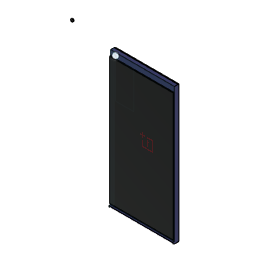
phone v1 (Autodesk Fusion 360 design; units mm, degrees)
Autodesk Fusion 360 part; units mm, degrees
sketch "Sketch1" plane through (0, 0, 0) normal (0, 1, 0) x (1, 0, 0)
  line L0 (-19.0423, -73.6284) -> (-12.0423, -73.6284)
  line L1 (-12.0423, -73.6284) -> (-12.0423, -58.6284)
  line L2 (-12.0423, -58.6284) -> (-19.0423, -58.6284)
  line L3 (-19.0423, -58.6284) -> (-19.0423, -73.6284)
  line L4 (-18.5, -73) -> (-16.5, -73)
  line L5 (-16.5, -73) -> (-16.5, -69)
  line L6 (-16.5, -69) -> (-18.5, -69)
  line L7 (-18.5, -69) -> (-18.5, -73)
  circle A0 centre (-17.5247, -72.1484) radius 0.6603
  circle A1 centre (-17.5247, -70.6133) radius 0.6107
  circle A2 centre (-18, -69.5) radius 0.2531
  circle A3 centre (-17, -69.5) radius 0.2276
  dimension "d1" = 7
  dimension "d2" = 15
  dimension "d3" = 2
  dimension "d4" = 4
  constraint horizontal L0
  constraint vertical L1
  constraint horizontal L2
  constraint vertical L3
  constraint horizontal L4
  constraint vertical L5
  constraint horizontal L6
  constraint vertical L7
  measures "d1" distance of L0.start L0.end
  measures "d2" distance of L0.start L2.end
  measures "d3" distance of L4.start L4.end
  measures "d4" distance of L4.start L6.end
extrude "Extrude1" add sketch "Sketch1" against normal blind 1 contours L0 L1 L2 L3 makes body 1
extrude "Extrude2" add sketch "Sketch1" along normal blind 0.5 separate body contours L4 L5 L6 L7 makes body 2
extrude "Extrude3" add sketch "Sketch1" along normal blind 1 contours A0 bodies 2
extrude "Extrude4" add sketch "Sketch1" along normal blind 0.75 contours A1 bodies 2
extrude "Extrude5" cut 1 faces at (-17.3264, 1, 72.3095) along direction (0, -1, 0) blind 0.25 on bodies 2 bodies 2
extrude "Extrude6" add sketch "Sketch1" along normal blind 0.65 contours A2 | A3 bodies 2
extrude "Extrude7" cut 1 faces at (-15.8615, -1, 62.0856) along direction (0, 1, 0) blind 0.2 on bodies 1 bodies 1
chamfer "Chamfer1" distance 0.1 angle 45 8 edges at (-15.5423, 0, 73.6284) (-19.0423, 0, 66.1284) (-12.0423, 0, 66.1284) (-15.5423, 0, 58.6284) (-16.5, 0.5, 71) (-18.5, 0.5, 71) (-17.5, 0.5, 69) (-17.5, 0.5, 73) 1 faces at (-17.8333, 0.1667, 73) on bodies 1 2
fillet "Fillet1" radius 0.25 2 edges at (-15.5423, -0.1, 73.6284) (-19.0423, -0.1, 66.1284) on bodies 1
fillet "Fillet2" radius 0.25 3 edges at (-12.1423, 0, 66.1284) (-15.5311, -0.1, 58.6284) (-15.5423, -0.8, 58.6284) on bodies 1
extrude "Extrude8" cut 1 faces at (-15.8615, -0.8, 62.2523) along direction (0, 1, 0) blind 0.2 on bodies 1 bodies 1
fillet "Fillet3" radius 0.03 4 edges at (-12.0559, -0.0864, 73.5993) (-12.0995, -0.0473, 73.5736) (-12.188, -0.0068, 73.5352) (-15.5941, 0, 73.5284) on bodies 1
sketch "Sketch2" plane through (-19.0423, 0, 0) normal (-1, 0, 0) x (0, -1, 0)
  line L0 (0.8, 58.8784) -> (0.6, 58.8784)
  line L1 (0.6, 58.8784) -> (0.6, 73.6284)
  line L2 (0.6, 73.6284) -> (0.2036, 73.6284)
  line L3 (0.2036, 73.6284) -> (0.2036, 58.6284)
  line L4 (0.2036, 58.6284) -> (0.55, 58.6284)
  arc A0 (0.55, 58.6284) -> (0.8, 58.8784) centre (0.55, 58.8784) ccw
sketch "Sketch3" plane through (-19.0423, 0, 0) normal (-1, 0, 0) x (0, -1, 0)
box "BoxPrimitive1" add length 14 width 7 height 1 placed x (0, 0, -1) y (-1, 0, 0) z (0, 1, 0) at (-3.7259, 0, 72.9723) separate body makes body 3
sketch "Sketch5" plane through (0, 0, 0) normal (0, -1, 0) x (1, 0, 0)
  line L0 (-10.7259, 58.9723) -> (-3.7259, 58.9723)
  line L1 (-3.7259, 58.9723) -> (-3.7259, 72.9723)
  line L2 (-3.7259, 72.9723) -> (-10.7259, 72.9723)
  line L3 (-10.7259, 72.9723) -> (-10.7259, 58.9723)
extrude "Extrude9" cut sketch "Sketch5" against normal blind 0.9 bodies 3
sketch "Sketch6" plane through (0, -0.6, 0) normal (0, -1, 0) x (1, 0, 0)
  line L0 (-19.0423, 58.8784) -> (-12.0423, 58.8784)
  line L1 (-12.0423, 58.8784) -> (-12.0423, 73.6284)
  line L2 (-12.0423, 73.6284) -> (-19.0423, 73.6284)
  line L3 (-19.0423, 73.6284) -> (-19.0423, 58.8784)
  line L4 (-18.5, 69) -> (-18.5, 73)
  line L5 (-18.5, 73) -> (-16.5, 73)
  line L6 (-16.5, 73) -> (-16.5, 69)
  line L7 (-16.5, 69) -> (-18.5, 69)
  circle A0 centre (-18.5, 73.3311) radius 0.2391
cylinder "CylinderPrimitive1" add diameter 0.294 height 0.1 placed x (1, 0, 0) y (0, 0, 1) z (0, -1, 0) at (-23.2082, -0.6, 74.3845) separate body makes body 4
move_body "Move1" bodies 3 to x (1, 0, 0) y (0, 1, 0) z (0, 0, 1) at (-8.2848, -1.6476, 0.122)
extrude "Extrude10" cut 2 faces at (-17.3925, 0.75, 70.4369) (-17.3264, 0.75, 72.3095) along direction (0, -1, 0) blind 0.4 on bodies 2 bodies 2
cylinder "CylinderPrimitive2" add diameter 1.131 height 0.1 placed x (1, 0, 0) y (0, 0, -1) z (0, 1, 0) at (-20.9, 0, 71.5) separate body makes body 5
cylinder "CylinderPrimitive3" add diameter 1.025 height 0.1 placed x (1, 0, 0) y (0, 0, -1) z (0, 1, 0) at (-21.3, 0, 70.1) separate body makes body 6
move_body "Move2" bodies 5 to x (1, 0, 0) y (0, 1, 0) z (0, 0, 1) at (3.3676, 0.4, 0.6625)
move_face "MoveFace1" by (-0.0333, 0.0779, 1.5703) 1 faces at (-21.2398, 0.1, 69.9482) on bodies 6
move_body "Move3" bodies 6 to x (1, 0, 0) y (0, 1, 0) z (0, 0, 1) at (3.7644, 0.2551, 0.5187)
cylinder "CylinderPrimitive4" add diameter 0.4 height 0.1 placed x (1, 0, 0) y (0, 0, -1) z (0, 1, 0) at (-20.6, 0, 69.7) separate body makes body 7
cylinder "CylinderPrimitive5" add diameter 0.283 height 0.1 placed x (1, 0, 0) y (0, 0, -1) z (0, 1, 0) at (-21.4, 0, 70.2) separate body makes body 8
move_body "Move4" bodies 8 to x (1, 0, 0) y (0, 1, 0) z (0, 0, 1) at (3.3792, 0.5652, -0.6952)
move_body "Move5" bodies 7 to x (1, 0, 0) y (0, 1, 0) z (0, 0, 1) at (3.592, 0.6, -0.2002)
